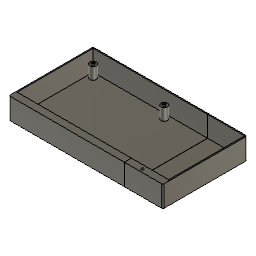
p4-screen-case (Autodesk Fusion 360 design; units mm, degrees)
part number: 2026-07-09-18-33-15-201
Autodesk Fusion 360 part; units mm, degrees
note: some values were not read from the file. Chosen so that the rebuilt part matches the saved one: which bodies a step acts on; that a step has no effect. Set by a fixed rule: which sketch regions a step uses.
sketch "Sketch1" plane through (0, 0, 0) normal (0, 0, 1) x (1, 0, 0)
  line L0 (0, 0) -> (256.5, 0)
  line L1 (256.5, 0) -> (256.5, 128.5)
  line L2 (256.5, 128.5) -> (0, 128.5)
  line L3 (0, 128.5) -> (0, 0)
  circle A0 centre (8, 8) radius 2.5
  circle A1 centre (128.25, 8) radius 2.5
  circle A2 centre (248.5, 8) radius 2.5
  circle A3 centre (8, 120.5) radius 2.5
  circle A4 centre (128.25, 120.5) radius 2.5
  circle A5 centre (248.5, 120.5) radius 2.5
  line L4 (-2, -2) -> (258.5, -2)
  line L5 (258.5, -2) -> (258.5, 128.5)
  line L6 (256.5, 130.5) -> (0, 130.5)
  line L7 (-2, 128.5) -> (-2, -2)
  circle A6 centre (128.25, 8) radius 4.5
  circle A7 centre (248.5, 8) radius 4.5
  circle A8 centre (248.5, 120.5) radius 4.5
  circle A9 centre (128.25, 120.5) radius 4.5
  circle A10 centre (8, 120.5) radius 4.5
  line L8 (0, -12) -> (256.5, -12)
  line L9 (-2, -10) -> (-2, -2)
  line L10 (258.5, -10) -> (258.5, -2)
  circle A11 centre (8, 8) radius 4.5
  circle A12 centre (8, 8) radius 5.5
  circle A13 centre (128.25, 8) radius 5.5
  circle A14 centre (248.5, 8) radius 5.5
  circle A15 centre (248.5, 120.5) radius 5.5
  circle A16 centre (128.25, 120.5) radius 5.5
  circle A17 centre (8, 120.5) radius 5.5
  circle A18 centre (218.5, -6.5) radius 2
  arc A19 (0, 130.5) -> (-2, 128.5) centre (0, 128.5) ccw
  arc A20 (-2, -10) -> (0, -12) centre (0, -10) ccw
  arc A21 (256.5, -12) -> (258.5, -10) centre (256.5, -10) ccw
  arc A22 (258.5, 128.5) -> (256.5, 130.5) centre (256.5, 128.5) ccw
  line L11 (193.4002, 130.5) -> (193.4002, -12)
  dimension "d1" = 256.5
  dimension "d2" = 128.5
  dimension "d9" = 5
  dimension "d10" = 8
  dimension "d11" = 8
  dimension "d12" = 5
  dimension "d13" = 8
  dimension "d14" = 5
  dimension "d15" = 8
  dimension "d16" = 8
  dimension "d17" = 5
  dimension "d18" = 8
  dimension "d19" = 8
  dimension "d20" = 5
  dimension "d21" = 8
  dimension "d22" = 5
  dimension "d23" = 8
  dimension "d24" = 8
  dimension "d31" = 2
  dimension "d32" = 2
  dimension "d33" = 2
  dimension "d34" = 2
  dimension "d35" = 2
  dimension "d37" = 2
  dimension "d38" = 1
  dimension "d39" = 1
  dimension "d40" = 1
  dimension "d41" = 1
  dimension "d42" = 1
  dimension "d43" = 1
  dimension "d44" = 4
  dimension "d45" = 40
  dimension "d46" = 5.5
  dimension "d66" = 2
  dimension "d67" = 2
  dimension "d68" = 2
  constraint horizontal L0
  constraint vertical L1
  constraint horizontal L2
  constraint vertical L3
  constraint coincident L0.start L3.end
  constraint perpendicular L4 L9
  constraint perpendicular L4 L10
  constraint tangent L6 A19
  constraint tangent L7 A19
  constraint tangent L8 A20
  constraint tangent L9 A20
  constraint tangent L10 A21
  constraint tangent L8 A21
  constraint tangent L5 A22
  constraint tangent L6 A22
  constraint equal A21 A22
  constraint coincident L6 L11.start
  constraint perpendicular L6 L11
  constraint coincident L8 L11.end
  measures "d1" distance of L0.start L0.end
  measures "d2" distance of L0.start L2.end
  measures "d9" diameter of A0
  measures "d10" distance of L3 A0.centre
  measures "d11" distance of L0 A0.centre
  measures "d12" diameter of A1
  measures "d13" distance of L0 A1.centre
  measures "d14" diameter of A2
  measures "d15" distance of L0 A2.centre
  measures "d16" distance of L1 A2.centre
  measures "d17" diameter of A3
  measures "d18" distance of L2 A3.centre
  measures "d19" distance of L3 A3.centre
  measures "d20" diameter of A4
  measures "d21" distance of L2 A4.centre
  measures "d22" diameter of A5
  measures "d23" distance of L1 A5.centre
  measures "d24" distance of L2 A5.centre
  measures "d44" diameter of A18
  measures "d45" distance of L10 A18.centre
  measures "d46" distance of L8 A18.centre
  measures "d66" radius of A19
  measures "d67" radius of A20
  measures "d68" radius of A21
extrude "Extrude11" cut sketch "Sketch1" along normal blind 20 contours A6 | A9 | A10 | A11
extrude "Extrude12" [no effect]
extrude "Extrude14" add sketch "Sketch1" along normal blind 36 separate body contours L0 L2 L3 L4 L6 L7 A19 L11 | L4 L8 L9 A20 L11 makes body 1
extrude "Extrude15" add sketch "Sketch1" along normal blind 21 separate body contours A6 | A9 | A10 | A11 | A12 | A13 | A16 | A17 makes body 2 at (13.4932, 7.7258, 14) makes body 3 at (133.7432, 7.7258, 14) makes body 4 at (13.4932, 120.2258, 14) makes body 5 at (133.7432, 120.2258, 14)
extrude "Extrude16" cut sketch "Sketch1" along normal blind 20 contours A6 | A9 | A10 | A11 bodies 2 3 4 5
extrude "Extrude17" add sketch "Sketch1" along normal blind 1 contours L0 L2 L3 L11 bodies 1 2 3 4 5
extrude "Extrude18" add sketch "Sketch1" along normal blind 1 separate body contours L0 L1 L2 L11 makes body 6
extrude "Extrude19" add sketch "Sketch1" along normal blind 36 contours L0 L1 L2 L4 L5 L6 A22 L11 | L4 L8 L10 A21 L11 bodies 6
extrude "Extrude20" add sketch "Sketch1" along normal blind 21 contours A7 | A8 | A14 | A15 bodies 6
extrude "Extrude21" cut sketch "Sketch1" along normal blind 20 contours A7 | A8 bodies 6
sketch "Sketch3" plane through (0, -12, 0) normal (0, -1, 0) x (1, 0, 0)
  line L0 (193.4002, 0) -> (256.5, 0)
  line L1 (256.5, 0) -> (256.5, 36)
  line L2 (256.5, 36) -> (193.4002, 36)
  line L3 (193.4002, 36) -> (193.4002, 0)
  line L4 (255, 36) -> (246, 36)
  line L5 (246, 0) -> (255, 0)
  line L6 (255, 0) -> (255, 36)
  line L7 (246, 35) -> (255, 35)
  line L8 (246, 1) -> (255, 1)
  line L9 (0, 0) -> (256.5, 0)
  line L10 (246, 0) -> (236, 0)
  line L11 (236, 36) -> (246, 36)
  line L12 (236, 36) -> (211, 36)
  line L13 (211, 36) -> (211, 1)
  line L14 (211, 1) -> (236, 1)
  line L15 (236, 35) -> (236, 36)
  line L16 (246, 35) -> (211, 35)
  line L17 (246, 1) -> (236, 1)
  line L18 (206, 6.8552) -> (206, 0)
  line L19 (206, 0) -> (196.9026, 0)
  line L20 (196.9026, 0) -> (196.9026, 6.8552)
  arc A0 (205.8979, 6.8552) -> (196.9026, 6.8552) centre (201.4002, 7) ccw
  line L21 (205.8979, 6.8552) -> (205.8979, 0)
  line L22 (246, 36) -> (246, 35)
  line L23 (246, 1) -> (246, 0)
  line L24 (236, 0) -> (236, 1)
  line L25 (236, 35) -> (236, 36)
  line L26 (246, 36) -> (246, 35)
  line L27 (246, 1) -> (246, 0)
  dimension "d85" = 1
  dimension "d86" = 1
  dimension "d91" = 9
  dimension "d92" = 7
  dimension "d97" = 10
  dimension "d98" = 25
  dimension "d99" = 35
  dimension "d108" = 8
  constraint horizontal L4
  constraint vertical L22
  constraint horizontal L5
  constraint vertical L6
  constraint coincident L0 L5.start
  constraint coincident L2 L4.start
  constraint perpendicular L7 L22
  constraint coincident L6 L7.end
  constraint perpendicular L8 L23
  constraint coincident L6 L8.end
  constraint horizontal L10
  constraint vertical L24
  constraint horizontal L11
  constraint vertical L26
  constraint horizontal L12
  constraint vertical L13
  constraint horizontal L14
  constraint vertical L15
  constraint coincident L13 L16.end
  constraint perpendicular L13 L16
  constraint coincident L14.end L24
  constraint perpendicular L17 L24
  constraint vertical L18
  constraint horizontal L19
  constraint vertical L20
  constraint coincident L9 L18.end
  constraint vertical L21
  constraint coincident L9 L21.end
  constraint coincident L16 L15.start
  constraint collinear L22 L23
  constraint collinear L24 L25
  constraint collinear L26 L27
  measures "d85" distance of L4 L7
  measures "d86" distance of L5 L8
  measures "d91" diameter of A0
  measures "d92" distance of A0.centre L9
  measures "d97" distance of L5.start L10.end
  measures "d98" distance of L11.start L12.end
  measures "d99" distance of L11.start L14.end
  measures "d108" distance of L3 A0.centre
extrude "Extrude22" [suppressed]
extrude "Extrude23" [suppressed]
extrude "Extrude24" [suppressed]
extrude "Extrude25" [suppressed]
extrude "Extrude26" [suppressed]
extrude "Extrude27" [suppressed]
extrude "Extrude28" [suppressed]
